gear-wheel v7 (Autodesk Fusion 360 design; units mm, degrees)
description: Spur Gear; Module: 0.4; Num Teeth: 30; Pressure Angle: 20.0; Backlash: 0.00 mm
Autodesk Fusion 360 part; units mm, degrees
sketch "スケッチ1" plane through (0, 0, 0) normal (0, 0, 1) x (1, 0, 0) in component "Spur Gear (30 teeth)"
  circle A0 centre (0, 0) radius 5.4692
  circle A1 centre (0, 0) radius 5
extrude "押し出し1" add sketch "スケッチ1" along normal blind 1 in component "Spur Gear (30 teeth)"
sketch "スケッチ2" plane through (0, 0, 0) normal (0, 0, 1) x (1, 0, 0) in component "Spur Gear (30 teeth)"
  spline S0 degree 3 poles (5.6254, -0.379) (5.6538, -0.3782) (5.7111, -0.3767) (5.7967, -0.3629) (5.8826, -0.3448) (5.9687, -0.3216) (6.0549, -0.2943) (6.141, -0.263) (6.2271, -0.2281) (6.3132, -0.1897) (6.3698, -0.1616) (6.3983, -0.1475) knots 0 0 0 0 0.008521 0.017175 0.025956 0.034865 0.043902 0.053065 0.062355 0.071773 0.081318 0.081318 0.081318 0.081318
  spline S1 degree 3 poles (5.6254, 0.379) (5.6538, 0.3782) (5.7111, 0.3767) (5.7967, 0.3629) (5.8826, 0.3448) (5.9687, 0.3216) (6.0549, 0.2943) (6.141, 0.263) (6.2271, 0.2281) (6.3132, 0.1897) (6.3698, 0.1616) (6.3983, 0.1475) knots 0 0 0 0 0.008521 0.017175 0.025956 0.034865 0.043902 0.053065 0.062355 0.071773 0.081318 0.081318 0.081318 0.081318
  arc A0 (6.3983, -0.1475) -> (6.3983, 0.1475) centre (0, 0) ccw
  line L0 (5.4469, -0.3676) -> (5.6254, -0.379)
  line L1 (5.4469, 0.3676) -> (5.6254, 0.379)
  line L2 (5.4469, -0.3676) -> (5.4469, 0.3676)
  point P0 (5.7105, -0.3748)
  point P1 (5.7961, -0.3623)
  point P2 (5.882, -0.3441)
  point P3 (5.9681, -0.3211)
  point P4 (6.0543, -0.2938)
  point P5 (6.1404, -0.2626)
  point P6 (6.2265, -0.2277)
  point P7 (6.3125, -0.1893)
  point P8 (5.7105, 0.3748)
  point P9 (5.7961, 0.3623)
  point P10 (5.882, 0.3441)
  point P11 (5.9681, 0.3211)
  point P12 (6.0543, 0.2938)
  point P13 (6.1404, 0.2626)
  point P14 (6.2265, 0.2277)
  point P15 (6.3125, 0.1893)
extrude "押し出し2" add sketch "スケッチ2" along normal blind 1 in component "Spur Gear (30 teeth)"
pattern_circular "C パターン1" count 30 over 360 about axis through (0, 0, 0) along (0, 0, 1) of "押し出し2" in component "Spur Gear (30 teeth)"
sketch "スケッチ3" plane through (0, 0, 0) normal (0, 0, 1) x (1, 0, 0) in component "Spur Gear (30 teeth)"
  circle A0 centre (0, 0) radius 6 construction
component "Spur Gear (30 teeth)" placed x (1, 0, 0) y (0, 1, 0) z (0, 0, 1) at (0, 0, 0)
